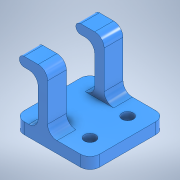
# Autodesk Inventor part: CableHook
Saved by Autodesk Inventor 2022 (Build 260153000, 153)
## iProperties
Created: 2022-02-22
Part Number: CableHook
Material: Generic
Document SubType Name: Modeling
Designer: Jorian Brusind
Density: 1 g/cm^3
Appearance: Cyan
Author: Jorian Brusind
Autodesk Inventor part; units mm, degrees
ref_plane "YZ Plane" through (0, 0, 0) normal (1, 0, 0) x (0, 1, 0)
ref_plane "XZ Plane" through (0, 0, 0) normal (0, 1, 0) x (-1, 0, 0)
ref_plane "XY Plane" through (0, 0, 0) normal (0, 0, 1) x (1, 0, 0)
sketch "Sketch1" plane through (0, 0, 0) normal (0, 1, 0) x (-1, 0, 0)
  line L0 (0, 0) -> (40, 0)
  line L1 (40, 0) -> (40, -40)
  line L2 (40, -40) -> (0, -40)
  line L3 (0, -40) -> (0, 0)
  line L4 (0, 0) -> (10, 0)
  line L5 (10, 0) -> (10, -10)
  line L6 (10, -10) -> (10, -30)
  circle A0 centre (10, -10) radius 3
  circle A1 centre (10, -30) radius 3
  dimension "d0" = 40
  dimension "d1" = 40
  dimension "d2" = 10
  dimension "d3" = 10
  dimension "d4" = 20
  dimension "d5" = 6
  dimension "d6" = 6
  constraints: 14 end point, 2 centre point, 2 coincident, 2 parallel, 2 perpendicular, 1 horizontal, 1 point on line, 1 vertical
  measures "d0" distance of L1.end L2.end
  measures "d1" distance of L0.end L1.end
  measures "d2" distance of L0.start L4.end
  measures "d3" distance of L4.end L5.end
  measures "d4" distance of L5.end L6.end
  measures "d5" diameter of A0
  measures "d6" diameter of A1
extrude "Extrusion1" add sketch "Sketch1" along normal blind 6
sketch "Sketch2" plane through (0, 6, 0) normal (0, 1, 0) x (1, 0, 0)
  line L0 (-40, 0) -> (0, 0) projected
  line L1 (-40, 0) -> (-25, 0)
  line L2 (-25, 0) -> (-25, 40)
  line L3 (0, 40) -> (-40, 40) projected
  line L4 (-25, 0) -> (-25, 5)
  line L5 (-25, 40) -> (-25, 35)
  line L6 (-22.5, 10) -> (-27.5, 10)
  line L7 (-27.5, 10) -> (-27.5, 0)
  line L8 (-27.5, 0) -> (-22.5, 0)
  line L9 (-22.5, 0) -> (-22.5, 10)
  line L10 (-22.5, 10) -> (-27.5, 0) construction
  line L11 (-27.5, 10) -> (-22.5, 0) construction
  line L12 (-22.5, 30) -> (-27.5, 30)
  line L13 (-27.5, 30) -> (-27.5, 40)
  line L14 (-27.5, 40) -> (-22.5, 40)
  line L15 (-22.5, 40) -> (-22.5, 30)
  line L16 (-22.5, 30) -> (-27.5, 40) construction
  line L17 (-27.5, 30) -> (-22.5, 40) construction
  dimension "d9" = 15
  dimension "d10" = 40
  dimension "d11" = 5
  dimension "d12" = 5
  dimension "d13" = 5
  dimension "d14" = 5
  dimension "d15" = 10
  constraints: 32 end point, 5 point on line, 4 midpoint, 4 parallel, 2 horizontal, 2 perpendicular
  measures "d9" distance of L0.start L1.end
  measures "d10" distance of L1.end L2.end
  measures "d11" distance of L1.end L4.end
  measures "d12" distance of L2.end L5.end
  measures "d13" distance of L8.end L7.end
  measures "d14" distance of L13.end L14.end
  measures "d15" distance of L12.end L13.end
extrude "Extrusion2" add sketch "Sketch2" along normal blind 30
sketch "Sketch3" plane through (-27.5, 6, -40) normal (-1, 0, 0) x (0, 0, 1)
  line L0 (40, 0) -> (40, 30) projected
  line L1 (40, 30) -> (30, 30)
  line L2 (30, 30) -> (30, 25)
  line L3 (30, 25) -> (40, 25)
  line L4 (40, 25) -> (40, 30)
  line L5 (10, 0) -> (10, 30) projected
  line L6 (10, 30) -> (0, 30)
  line L7 (0, 30) -> (0, 25)
  line L8 (0, 25) -> (10, 25)
  line L9 (10, 25) -> (10, 30)
  point P0 (40, -6)
  dimension "d18" = 10
  dimension "d19" = 5
  dimension "d20" = 10
  dimension "d21" = 5
  constraints: 16 end point, 4 parallel, 2 horizontal, 2 perpendicular
  measures "d18" distance of L3.end L2.end
  measures "d19" distance of L2.end L1.end
  measures "d20" distance of L8.end L7.end
  measures "d21" distance of L7.end L6.end
extrude "Extrusion3" add sketch "Sketch3" along normal blind 10
fillet "Fillet1" radius 5 6 edges at (-22.5, 36, -5) (-22.5, 36, -35) (-22.5, 6, -5) (-22.5, 6, -35) (-27.5, 31, -5) (-27.5, 31, -35)
fillet "Fillet2" radius 5 2 edges at (-27.5, 6, -5) (-27.5, 6, -35)
fillet "Fillet3" radius 5 4 edges at (-40, 3, -40) (-40, 3, 0) (0, 3, -40) (0, 3, 0)
fillet "Fillet4" radius 2.5 4 edges at (-37.5, 31, -5) (-37.5, 36, -5) (-37.5, 36, -35) (-37.5, 31, -35)
body "Solid1"
